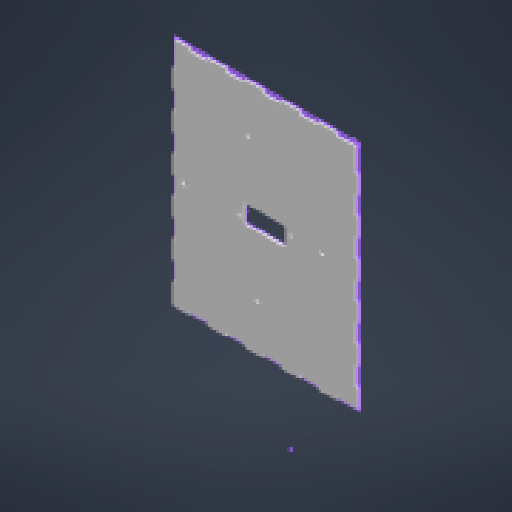
# Autodesk Inventor part: part5
Saved by Autodesk Inventor 2027.1 (Build 311270010, 270A)
## iProperties
Created: 2026-10-07
Part Number: part5
Material: Generic
Document SubType Name: Modeling
Designer: daniel
Density: 1 g/cm^3
Appearance: Default
Mass: 142.908 g
Surface Area: 989.489 cm^2
Volume: 142.908 cm^3
Author: daniel
Autodesk Inventor part; units mm, degrees
ref_plane "YZ Plane" through (0, 0, 0) normal (1, 0, 0) x (0, 1, 0)
ref_plane "XZ Plane" through (0, 0, 0) normal (0, 1, 0) x (-1, 0, 0)
ref_plane "XY Plane" through (0, 0, 0) normal (0, 0, 1) x (1, 0, 0)
sketch "Sketch1" plane through (0, 0, 0) normal (0, 0, 1) x (1, 0, 0)
  line L0 (81.6094, 169.8435) -> (-118.3906, 169.8435)
  line L1 (-118.3906, 169.8435) -> (-118.3906, -80.1565)
  line L2 (-118.3906, -80.1565) -> (81.6094, -80.1565)
  line L3 (81.6094, -80.1565) -> (81.6094, 169.8435)
  line L4 (81.6094, 169.8435) -> (58.6094, 169.8435)
  line L5 (58.6094, 169.8435) -> (58.6094, 166.8435)
  line L6 (58.6094, 166.8435) -> (81.6094, 166.8435)
  line L7 (81.6094, 166.8435) -> (81.6094, 169.8435)
  line L8 (58.6094, 166.8435) -> (38.6094, 166.8435)
  line L9 (38.6094, 166.8435) -> (38.6094, 169.8435)
  line L10 (38.6094, 169.8435) -> (58.6094, 169.8435)
  line L11 (58.6094, 169.8435) -> (58.6094, 166.8435)
  line L12 (38.6094, 166.8435) -> (18.7094, 166.8435)
  line L13 (18.7094, 166.8435) -> (18.7094, 169.8435)
  line L14 (18.7094, 169.8435) -> (38.6094, 169.8435)
  line L15 (38.6094, 169.8435) -> (38.6094, 166.8435)
  line L16 (18.7094, 166.8435) -> (-1.2906, 166.8435)
  line L17 (-1.2906, 166.8435) -> (-1.2906, 169.8435)
  line L18 (-1.2906, 169.8435) -> (18.7094, 169.8435)
  line L19 (18.7094, 169.8435) -> (18.7094, 166.8435)
  line L20 (-1.2906, 166.8435) -> (-21.1906, 166.8435)
  line L21 (-21.1906, 166.8435) -> (-21.1906, 169.8435)
  line L22 (-21.1906, 169.8435) -> (-1.2906, 169.8435)
  line L23 (-1.2906, 169.8435) -> (-1.2906, 166.8435)
  line L24 (-21.1906, 166.8435) -> (-41.1906, 166.8435)
  line L25 (-41.1906, 166.8435) -> (-41.1906, 169.8435)
  line L26 (-41.1906, 169.8435) -> (-21.1906, 169.8435)
  line L27 (-21.1906, 169.8435) -> (-21.1906, 166.8435)
  line L28 (-111.1906, 169.8435) -> (-91.1906, 169.8435)
  line L29 (-91.1906, 169.8435) -> (-118.3906, 169.8435)
  line L30 (-118.3906, 169.8435) -> (-118.3906, 166.8435)
  line L31 (-118.3906, 166.8435) -> (-115.3906, 166.8435)
  line L32 (-118.3906, 142.8435) -> (-118.3906, 166.8435)
  line L33 (-118.3906, 169.8435) -> (-115.3906, 169.8435)
  line L34 (-115.3906, 169.8435) -> (-115.3906, 142.2435)
  line L35 (-115.3906, 142.2435) -> (-118.3906, 142.2435)
  line L36 (-118.3906, 142.2435) -> (-118.3906, 169.8435)
  line L37 (-118.3906, 142.2435) -> (-115.3906, 142.2435)
  line L38 (-115.3906, 142.2435) -> (-115.3906, 122.2435)
  line L39 (-115.3906, 122.2435) -> (-118.3906, 122.2435)
  line L40 (-118.3906, 122.2435) -> (-118.3906, 142.2435)
  line L41 (-115.3906, 122.2435) -> (-118.3906, 122.2435)
  line L42 (-118.3906, 122.2435) -> (-118.3906, 102.3435)
  line L43 (-118.3906, 102.3435) -> (-115.3906, 102.3435)
  line L44 (-115.3906, 102.3435) -> (-115.3906, 122.2435)
  line L45 (-118.3906, 102.3435) -> (-115.3906, 102.3435)
  line L46 (-115.3906, 102.3435) -> (-115.3906, 82.3435)
  line L47 (-115.3906, 82.3435) -> (-118.3906, 82.3435)
  line L48 (-118.3906, 82.3435) -> (-118.3906, 102.3435)
  line L49 (-118.3906, 82.3435) -> (-115.3906, 82.3435)
  line L50 (-115.3906, 82.3435) -> (-115.3906, 62.4435)
  line L51 (-115.3906, 62.4435) -> (-118.3906, 62.4435)
  line L52 (-118.3906, 62.4435) -> (-118.3906, 82.3435)
  line L53 (-118.3906, 62.4435) -> (-115.3906, 62.4435)
  line L54 (-115.3906, 62.4435) -> (-115.3906, 42.4435)
  line L55 (-115.3906, 42.4435) -> (-118.3906, 42.4435)
  line L56 (-118.3906, 42.4435) -> (-118.3906, 62.4435)
  line L57 (-118.3906, 42.4435) -> (-115.3906, 42.4435)
  line L58 (-115.3906, 42.4435) -> (-115.3906, 22.5435)
  line L59 (-115.3906, 22.5435) -> (-118.3906, 22.5435)
  line L60 (-118.3906, 22.5435) -> (-118.3906, 42.4435)
  line L61 (-118.3906, 22.5435) -> (-115.3906, 22.5435)
  line L62 (-115.3906, 22.5435) -> (-115.3906, 2.5435)
  line L63 (-115.3906, 2.5435) -> (-118.3906, 2.5435)
  line L64 (-118.3906, 2.5435) -> (-118.3906, 22.5435)
  line L65 (-118.3906, 2.5435) -> (-115.3906, 2.5435)
  line L66 (-115.3906, 2.5435) -> (-115.3906, -17.3565)
  line L67 (-115.3906, -17.3565) -> (-118.3906, -17.3565)
  line L68 (-118.3906, -17.3565) -> (-118.3906, 2.5435)
  line L69 (-118.3906, -17.3565) -> (-115.3906, -17.3565)
  line L70 (-115.3906, -17.3565) -> (-115.3906, -37.3565)
  line L71 (-115.3906, -37.3565) -> (-118.3906, -37.3565)
  line L72 (-118.3906, -37.3565) -> (-118.3906, -17.3565)
  line L73 (-118.3906, -37.3565) -> (-115.3906, -37.3565)
  line L74 (-115.3906, -37.3565) -> (-115.3906, -57.2565)
  line L75 (-115.3906, -57.2565) -> (-118.3906, -57.2565)
  line L76 (-118.3906, -57.2565) -> (-118.3906, -37.3565)
  line L77 (-118.3906, -57.2565) -> (-115.3906, -57.2565)
  line L78 (-115.3906, -57.2565) -> (-115.3906, -77.2565)
  line L79 (-115.3906, -77.2565) -> (-118.3906, -77.2565)
  line L80 (-118.3906, -77.2565) -> (-118.3906, -57.2565)
  line L81 (81.6094, 169.8435) -> (81.6094, -80.1565)
  line L82 (81.6094, 169.8435) -> (81.6094, 166.8435)
  line L83 (81.6094, 166.8435) -> (78.6094, 166.8435)
  line L84 (81.6094, 169.8435) -> (78.6094, 169.8435)
  line L85 (78.6094, 169.8435) -> (78.6094, 142.2435)
  line L86 (81.6094, 142.2435) -> (81.6094, 169.8435)
  line L87 (81.6094, 142.8435) -> (81.6094, 166.8435)
  line L88 (78.6094, 142.2435) -> (81.6094, 142.2435)
  line L89 (81.6094, 142.2435) -> (78.6094, 142.2435)
  line L90 (78.6094, 142.2435) -> (78.6094, 122.2435)
  line L91 (78.6094, 122.2435) -> (81.6094, 122.2435)
  line L92 (78.6094, 122.2435) -> (81.6094, 122.2435)
  line L93 (81.6094, 122.2435) -> (81.6094, 142.2435)
  line L94 (78.6094, 102.3435) -> (78.6094, 122.2435)
  line L95 (81.6094, 122.2435) -> (81.6094, 102.3435)
  line L96 (81.6094, 102.3435) -> (78.6094, 102.3435)
  line L97 (81.6094, 102.3435) -> (78.6094, 102.3435)
  line L98 (78.6094, 102.3435) -> (78.6094, 82.3435)
  line L99 (81.6094, 82.3435) -> (81.6094, 102.3435)
  line L100 (78.6094, 82.3435) -> (81.6094, 82.3435)
  line L101 (81.6094, 82.3435) -> (78.6094, 82.3435)
  line L102 (78.6094, 82.3435) -> (78.6094, 62.4435)
  line L103 (81.6094, 62.4435) -> (81.6094, 82.3435)
  line L104 (78.6094, 62.4435) -> (81.6094, 62.4435)
  line L105 (81.6094, 62.4435) -> (78.6094, 62.4435)
  line L106 (78.6094, 62.4435) -> (78.6094, 42.4435)
  line L107 (81.6094, 42.4435) -> (81.6094, 62.4435)
  line L108 (78.6094, 42.4435) -> (81.6094, 42.4435)
  line L109 (81.6094, 42.4435) -> (78.6094, 42.4435)
  line L110 (81.6094, 22.5435) -> (81.6094, 42.4435)
  line L111 (78.6094, 42.4435) -> (78.6094, 22.5435)
  line L112 (78.6094, 2.5435) -> (81.6094, 2.5435)
  line L113 (81.6094, 2.5435) -> (78.6094, 2.5435)
  line L114 (81.6094, 22.5435) -> (78.6094, 22.5435)
  line L115 (81.6094, 2.5435) -> (81.6094, 22.5435)
  line L116 (78.6094, 22.5435) -> (78.6094, 2.5435)
  line L117 (78.6094, 2.5435) -> (78.6094, -17.3565)
  line L118 (81.6094, -17.3565) -> (81.6094, 2.5435)
  line L119 (78.6094, 22.5435) -> (81.6094, 22.5435)
  line L120 (78.6094, -17.3565) -> (78.6094, -37.3565)
  line L121 (78.6094, -17.3565) -> (81.6094, -17.3565)
  line L122 (81.6094, -37.3565) -> (81.6094, -17.3565)
  line L123 (78.6094, -57.2565) -> (81.6094, -57.2565)
  line L124 (81.6094, -57.2565) -> (78.6094, -57.2565)
  line L125 (78.6094, -37.3565) -> (78.6094, -57.2565)
  line L126 (81.6094, -57.2565) -> (81.6094, -37.3565)
  line L127 (78.6094, -77.2565) -> (81.6094, -77.2565)
  line L128 (78.6094, -57.2565) -> (78.6094, -77.2565)
  line L129 (81.6094, -77.2565) -> (81.6094, -57.2565)
  line L130 (81.6094, -17.3565) -> (78.6094, -17.3565)
  line L131 (78.6094, -37.3565) -> (81.6094, -37.3565)
  line L132 (81.6094, -37.3565) -> (78.6094, -37.3565)
  line L133 (81.6094, -80.1565) -> (58.6094, -80.1565)
  line L134 (58.6094, -80.1565) -> (58.6094, -77.1565)
  line L135 (58.6094, -77.1565) -> (81.6094, -77.1565)
  line L136 (81.6094, -77.1565) -> (81.6094, -80.1565)
  line L137 (58.6094, -80.1565) -> (38.6094, -80.1565)
  line L138 (38.6094, -80.1565) -> (38.6094, -77.1565)
  line L139 (38.6094, -77.1565) -> (58.6094, -77.1565)
  line L140 (58.6094, -77.1565) -> (58.6094, -80.1565)
  line L141 (38.6094, -80.1565) -> (18.7094, -80.1565)
  line L142 (18.7094, -80.1565) -> (18.7094, -77.1565)
  line L143 (18.7094, -77.1565) -> (38.6094, -77.1565)
  line L144 (38.6094, -77.1565) -> (38.6094, -80.1565)
  line L145 (18.7094, -80.1565) -> (-1.2906, -80.1565)
  line L146 (-1.2906, -80.1565) -> (-1.2906, -77.1565)
  line L147 (-1.2906, -77.1565) -> (18.7094, -77.1565)
  line L148 (18.7094, -77.1565) -> (18.7094, -80.1565)
  line L149 (-1.2906, -77.1565) -> (-21.1906, -77.1565)
  line L150 (-21.1906, -77.1565) -> (-21.1906, -80.1565)
  line L151 (-21.1906, -80.1565) -> (-1.2906, -80.1565)
  line L152 (-1.2906, -80.1565) -> (-1.2906, -77.1565)
  line L153 (-21.1906, -80.1565) -> (-41.1906, -80.1565)
  line L154 (-41.1906, -80.1565) -> (-41.1906, -77.1565)
  line L155 (-41.1906, -77.1565) -> (-21.1906, -77.1565)
  line L156 (-21.1906, -77.1565) -> (-21.1906, -80.1565)
  line L157 (-41.1906, -77.1565) -> (-111.0906, -77.1565)
  line L158 (-61.0906, -80.1565) -> (-41.1906, -80.1565)
  line L159 (-41.1906, -80.1565) -> (-41.1906, -77.1565)
  line L160 (-111.0906, -77.1565) -> (-118.3906, -77.1565)
  line L161 (-118.3906, -77.1565) -> (-118.3906, -80.1565)
  line L162 (-118.3906, -80.1565) -> (-61.0906, -80.1565)
  line L163 (-61.0906, -80.1565) -> (-81.0906, -80.1565)
  line L164 (-81.0906, -80.1565) -> (-81.0906, -77.1565)
  line L165 (-81.0906, -77.1565) -> (-61.0906, -77.1565)
  line L166 (-61.0906, -77.1565) -> (-61.0906, -80.1565)
  line L167 (-81.0906, -77.1565) -> (-100.9906, -77.1565)
  line L168 (-100.9906, -77.1565) -> (-100.9906, -80.1565)
  line L169 (-100.9906, -80.1565) -> (-81.0906, -80.1565)
  line L170 (-81.0906, -80.1565) -> (-81.0906, -77.1565)
  line L171 (-41.1906, 166.8435) -> (-61.0906, 166.8435)
  line L172 (-61.0906, 166.8435) -> (-61.0906, 169.8435)
  line L173 (-61.0906, 169.8435) -> (-41.1906, 169.8435)
  line L174 (-41.1906, 169.8435) -> (-41.1906, 166.8435)
  line L175 (-61.0906, 166.8435) -> (-81.0906, 166.8435)
  line L176 (-81.0906, 166.8435) -> (-81.0906, 169.8435)
  line L177 (-81.0906, 169.8435) -> (-61.0906, 169.8435)
  line L178 (-61.0906, 169.8435) -> (-61.0906, 166.8435)
  line L179 (-81.0906, 166.8435) -> (-100.9906, 166.8435)
  line L180 (-100.9906, 166.8435) -> (-100.9906, 169.8435)
  line L181 (-100.9906, 169.8435) -> (-81.0906, 169.8435)
  line L182 (-81.0906, 169.8435) -> (-81.0906, 166.8435)
  line L183 (-100.9906, 166.8435) -> (-118.3906, 166.8435)
  line L184 (-118.3906, 166.8435) -> (-118.3906, 169.8435)
  line L185 (-118.3906, 169.8435) -> (-100.9906, 169.8435)
  line L186 (-100.9906, 169.8435) -> (-100.9906, 166.8435)
  line L187 (-40.8906, 34.9435) -> (4.1094, 34.9435)
  line L188 (4.1094, 34.9435) -> (4.1094, 54.7435)
  line L189 (4.1094, 54.7435) -> (-40.8906, 54.7435)
  line L190 (-40.8906, 54.7435) -> (-40.8906, 34.9435)
  point P0 (0, 0)
  point P1 (6.6094, -153.3151)
  point P2 (74.4094, 169.8435)
  point P3 (-115.3906, 2.5435)
  point P4 (-115.3906, -77.1565)
  point P5 (78.6094, -77.1565)
  point P6 (38.6094, 169.8435)
  point P7 (-118.3906, -57.2565)
  point P8 (-118.3906, -77.2565)
  point P9 (-118.3906, -17.3565)
  point P10 (-118.3906, -37.3565)
  point P11 (-118.3906, 22.5435)
  point P12 (-118.3906, 2.5435)
  point P13 (-118.3906, 42.4435)
  point P14 (-118.3906, 142.2435)
  point P15 (-118.3906, 122.2435)
  point P16 (-115.3906, -37.3565)
  point P17 (-118.3906, -77.1565)
  point P18 (-118.3906, 42.4435)
  point P19 (-118.3906, 22.5435)
  point P20 (-118.3906, 2.5435)
  point P21 (-118.3906, -17.3565)
  point P22 (-115.3906, 169.8435)
  point P23 (-118.3906, 44.8435)
  point P24 (-40.8906, 44.8435)
  point P25 (-31.1906, -80.1565)
  dimension "d0" = 200
  dimension "d1" = 250
  dimension "d2" = 23
  dimension "d3" = 3
  dimension "d4" = 20
  dimension "d5" = 19.9
  dimension "d6" = 20
  dimension "d7" = 19.9
  dimension "d8" = 20
  dimension "d9" = 3
  dimension "d10" = 27.6
  dimension "d11" = 3
  dimension "d12" = 20
  dimension "d13" = 19.9
  dimension "d14" = 20
  dimension "d15" = 19.9
  dimension "d16" = 20
  dimension "d17" = 19.9
  dimension "d18" = 20
  dimension "d19" = 19.9
  dimension "d20" = 20
  dimension "d21" = 3
  dimension "d22" = 19.9
  dimension "d23" = 20
  dimension "d24" = 23
  dimension "d25" = 3
  dimension "d26" = 20
  dimension "d27" = 19.9
  dimension "d28" = 19.9
  dimension "d29" = 19.9
  dimension "d32" = 20
  dimension "d33" = 19.9
  dimension "d34" = 19.9
  dimension "d35" = 20
  dimension "d36" = 19.9
  dimension "d37" = 45
  dimension "d38" = 19.8
  dimension "d39" = 77.5
  dimension "d40" = 115.1
  constraints: 376 end point, 64 parallel, 36 horizontal, 33 perpendicular, 26 point on line, 2 midpoint, 20 other
  measures "d0" distance of L81.end L2.start
  measures "d1" distance of L2.start point (-118.391, 169.844)
  measures "d2" distance of L7.start L6.start
  measures "d3" distance of L6.start L4.end
  measures "d4" distance of L9.end L11.start
  measures "d5" distance of L14.start L14.end
  measures "d6" distance of L18.start L19.start
  measures "d7" distance of L21.end L22.end
  measures "d8" distance of L25.end L27.start
  measures "d9" distance of L34.end L36.start
  measures "d10" distance of L33.end L34.end
  measures "d11" distance of L38.end L39.end
  measures "d12" distance of L37.end L38.end
  measures "d13" distance of L43.start L41.end
  measures "d14" distance of L45.end L47.start
  measures "d15" distance of L49.end L50.end
  measures "d16" distance of L53.end L55.start
  measures "d17" distance of L57.end L59.start
  measures "d18" distance of L61.end L62.end
  measures "d19" distance of L65.end L67.start
  measures "d20" distance of L69.end L70.end
  measures "d21" distance of L74.end L76.start
  measures "d22" distance of L73.end L74.end
  measures "d23" distance of L77.end L78.end
  measures "d24" distance of L135.start L136.start
  measures "d25" distance of L133.end L135.start
  measures "d26" distance of L138.end L140.start
  measures "d27" distance of L143.start L144.start
  measures "d28" distance of L152.start L151.start
  measures "d29" distance of L159.start L158.start
  measures "d32" distance of L164.end L165.end
  measures "d33" distance of L169.end L168.end
  measures "d34" distance of L172.end L173.end
  measures "d35" distance of L176.end L177.end
  measures "d36" distance of L180.end L181.end
  measures "d37" distance of L189.end L188.end
  measures "d38" distance of L188.end L187.end
  measures "d39" distance of point (-118.391, 44.844) point (-40.891, 44.844)
  measures "d40" distance from line of point (-31.191, -80.156) L187
extrude "Extrusion1" add sketch "Sketch1" along normal blind 3 contours L5 L8 L9 L0 | L85 L90 L94 L98 L102 L106 L111 L116 L117 L120 L125 L128 L135 L139 L143 L147 L149 L155 L157 L160 L78 L74 L70 L66 L62 L58 L54 L50 L46 L44 L38 L34 L183 L179 L175 L171 L24 L20 L16 L12 L8 L6 | L88 L3 L91 L90 | L13 L16 L17 L0 | L96 L3 L100 L98 | L21 L24 L25 L0 | L104 L3 L108 L106 | L172 L175 L176 L0 | L114 L3 L112 L116 | L180 L183 L34 L0 | L121 L3 L131 L120 | L38 L39 L1 L35 | L123 L3 L135 L128 | L46 L47 L1 L43 | L134 L2 L138 L139 | L54 L55 L1 L51 | L142 L2 L146 L147 | L62 L63 L1 L59 | L150 L2 L154 L155 | L70 L71 L1 L67 | L166 L2 L164 L157 | L78 L160 L1 L75 | L168 L2 L1 L79 L78 L160 L157 | L78 L79 L1 L160 | L190 L189 L188 L187
extrude "Extrusion2" cut sketch "Sketch1" along normal blind 3 contours L190 L189 L188 L187
sketch "Sketch2" plane through (0, 0, 3) normal (0, 0, 1) x (1, 0, 0)
  circle A0 centre (-31.2906, 44.8435) radius 75
  line L0 (-31.2906, 44.8435) -> (56.203, 50.348)
  line L1 (56.203, 50.348) -> (-118.9373, 39.3294)
  line L2 (-31.2906, 44.8435) -> (-24.9201, -56.4117)
  line L3 (-31.2906, 44.8435) -> (70.1649, 44.8435) construction
  line L4 (-24.9201, -56.4117) -> (-36.9493, 134.7868)
  circle A1 centre (43.5614, 49.5527) radius 2.5
  circle A2 centre (-106.1426, 40.1344) radius 2.5
  circle A3 centre (-35.9999, 119.6955) radius 2.5
  circle A4 centre (-26.5813, -30.0085) radius 2.5
  line L5 (4.1094, 34.9435) -> (-40.8906, 34.9435) projected
  line L6 (-40.8906, 54.7435) -> (4.1094, 54.7435) projected
  line L7 (4.1094, 34.9435) -> (-40.8906, 34.9435)
  line L8 (-40.8906, 34.9435) -> (-40.8906, 54.7435)
  line L9 (-40.8906, 54.7435) -> (4.1094, 54.7435)
  line L10 (4.1094, 54.7435) -> (4.1094, 34.9435)
  line L11 (-40.8906, 34.9435) -> (-40.8906, 54.7435) projected
  circle A5 centre (-31.2906, 44.8435) radius 1.6
  point P0 (0, 0)
  dimension "d43" = 150
  dimension "d44" = 86.4
  dimension "d45" = 5
  dimension "d46" = 5
  dimension "d47" = 5
  dimension "d48" = 5
  dimension "d49" = 9.9
  dimension "d50" = 9.6
  dimension "d51" = 3.2
  constraints: 18 end point, 6 centre point, 6 point on line, 4 point on circle, 2 horizontal, 2 parallel, 1 coincident, 1 equal length, 1 perpendicular
  measures "d43" diameter of A0
  measures "d44" angle of L2 L3
  measures "d45" diameter of A1
  measures "d46" diameter of A2
  measures "d47" diameter of A3
  measures "d48" diameter of A4
  measures "d49" distance from line of L6 L0.start
  measures "d50" distance from line of L11 L0.start
  measures "d51" diameter of A5
extrude "Extrusion3" cut sketch "Sketch2" against normal blind 3 contours A1 L0 A0 | A0 L0 A1 | A4 L2 A0 | A0 L2 A4 | L0 A1 A0 | A0 A1 L0 | L2 A4 A0 | A0 A4 L2 | A3 L4 A0 | A0 L4 A3 | A2 L1 A0 | A0 L1 A2 | L4 A3 A0 | A0 A3 L4 | L1 A2 A0 | A0 A2 L1
sketch "Sketch3" plane through (0, 0, 3) normal (0, 0, 1) x (1, 0, 0)
  circle A0 centre (-45.8906, 40.9435) radius 2
  circle A1 centre (9.6094, 48.7435) radius 2
  line L0 (-40.8906, 34.9435) -> (-40.8906, 54.7435) projected
  line L1 (4.1094, 54.7435) -> (4.1094, 34.9435) projected
  line L2 (-40.8906, 54.7435) -> (4.1094, 54.7435) projected
  line L3 (4.1094, 34.9435) -> (-40.8906, 34.9435) projected
  point P0 (0, 0)
  dimension "d54" = 4
  dimension "d55" = 4
  dimension "d56" = 5
  dimension "d57" = 5.5
  dimension "d58" = 6
  dimension "d59" = 6
  constraints: 2 centre point
  measures "d54" diameter of A0
  measures "d55" diameter of A1
  measures "d56" distance from line of A0.centre L0
  measures "d57" distance from line of A1.centre L1
  measures "d58" distance from line of L2 A1.centre
  measures "d59" distance from line of L3 A0.centre
extrude "Extrusion4" cut sketch "Sketch3" against normal blind 3 contours A0 | A1
equation "\"d39\" = -0.5 * d37 + 0.5 * d0"
equation "\"d40\" = -0.5 * d38 + 0.5 * d1"
body "Solid1"
